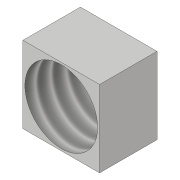
# Autodesk Inventor part: NUT SMALL
Saved by Autodesk Inventor 2019 (Build 230136000, 136)
## iProperties
Created: 2019-10-08
Part Number: NUT SMALL
Material: Generic
Document SubType Name: Modeling
Designer: Admin
Density: 1 g/cm^3
Appearance: Default
Author: Admin
Autodesk Inventor part; units mm, degrees
ref_plane "YZ Plane" through (0, 0, 0) normal (1, 0, 0) x (0, 1, 0)
ref_plane "XZ Plane" through (0, 0, 0) normal (0, 1, 0) x (-1, 0, 0)
ref_plane "XY Plane" through (0, 0, 0) normal (0, 0, 1) x (1, 0, 0)
sketch "Sketch1" plane through (0, 0, 0) normal (0, 0, 1) x (1, 0, 0)
  line L0 (0, 0) -> (2, 0)
  line L1 (2, 0) -> (2, 2)
  line L2 (2, 2) -> (0, 2)
  line L3 (0, 2) -> (0, 0)
  dimension "d0" = 2
  dimension "d1" = 2
  constraints: 8 end point, 2 parallel, 1 horizontal, 1 perpendicular
  measures "d0" distance of L2.end L1.end
  measures "d1" distance of L1.end L0.end
extrude "Extrusion1" add sketch "Sketch1" along normal blind 1.5
sketch "Sketch2" plane through (0, 0, 1.5) normal (0, 0, 1) x (1, 0, 0)
  line L0 (2, 2) -> (0, 2) projected
  line L1 (1, 2) -> (1, 0)
  line L2 (0, 0) -> (2, 0) projected
  circle A0 centre (1, 1) radius 0.95
  dimension "d4" = 1.9
  constraints: 3 midpoint, 2 end point, 1 centre point
  measures "d4" diameter of A0
extrude "Extrusion2" cut sketch "Sketch2" along normal through all both and the other way through all
thread "Thread1" size "M2x0.4" class "6H" standard "ANSI Metric M Profile" full length
body "Solid1"
